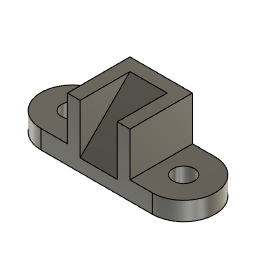
A2 (Autodesk Fusion 360 design; units mm, degrees)
Autodesk Fusion 360 part; units mm, degrees
sketch "Sketch2" plane through (0, 0, 0) normal (0, 0, 1) x (1, 0, 0)
  line L0 (57, -32) -> (-57, -32)
  line L1 (-57, 32) -> (57, 32)
  circle A0 centre (57, 0) radius 11
  circle A1 centre (-57, 0) radius 11
  arc A2 (-57, 32) -> (-57, -32) centre (-57, 0) ccw
  arc A3 (57, -32) -> (57, 32) centre (57, 0) ccw
  dimension "d15" = 114
  dimension "d17" = 32
  dimension "d18" = 32
  dimension "d19" = 22
  dimension "d20" = 22
  dimension "d21" = 114
  constraint horizontal L0
  constraint parallel L0 L1
  constraint concentric A0 A3
  constraint concentric A1 A2
  measures "d15" distance of L1.start L1.end
  measures "d17" radius of A3
  measures "d18" radius of A2
  measures "d19" diameter of A0
  measures "d20" diameter of A1
  measures "d21" distance of A0.centre A1.centre
extrude "Extrude1" add sketch "Sketch2" along normal blind 19
sketch "Sketch3" plane through (0, 0, 0) normal (0, 1, 0) x (1, 0, 0)
  line L0 (-30, 0) -> (34, 0)
  line L1 (34, 0) -> (34, -64)
  line L2 (34, -64) -> (-30, -64)
  line L3 (-30, -64) -> (-30, 0)
  dimension "d24" = 64
  dimension "d25" = 64
  constraint horizontal L0
  constraint vertical L1
  constraint horizontal L2
  constraint vertical L3
  measures "d24" distance of L0.start L0.end
  measures "d25" distance of L0.start L2.end
extrude "Extrude2" add sketch "Sketch3" along normal mid plane 64
shell "Shell1" thickness 13 removed faces 5 at (-8.6667, 32, 34) at (72.3041, 28.1031, 12.6667) at (12.6667, -32, 34) at (-77.5692, -24.5134, 12.6667) at (12.6667, -10.6667, 64)
sketch "Sketch4" plane through (0, 32, 0) normal (0, 1, 0) x (-1, 0, 0)
  line L0 (-21, 13) -> (-21, 64)
  line L1 (-21, 64) -> (-34, 64)
  line L2 (-34, 64) -> (-34, 19)
  line L3 (-34, 19) -> (-57, 19)
  line L4 (-57, 19) -> (-57, 0)
  line L5 (-57, 0) -> (57, 0)
  line L6 (57, 0) -> (57, 19)
  line L7 (57, 19) -> (30, 19)
  line L8 (30, 19) -> (30, 64)
  line L9 (30, 64) -> (17, 64)
  line L10 (17, 64) -> (17, 13)
  line L11 (17, 13) -> (-21, 13)
  line L12 (-21, 64) -> (17, 64)
  line L13 (17, 64) -> (17, 13)
  line L14 (17, 13) -> (-21, 13)
  line L15 (-21, 13) -> (-21, 64)
  constraint horizontal L12
  constraint vertical L13
  constraint horizontal L14
  constraint vertical L15
  constraint coincident L10.end L11.start
  constraint coincident L0.end L1.start
extrude "Extrude3" add sketch "Sketch4" against normal blind 13 contours L0 L10 L11 L12 L13 L14 L15
scale "Scale1" factor 0.887488 about (-17, -32, 64) bodies 1
sketch "Sketch8" plane through (16.7245, 0, 0) normal (-1, 0, 0) x (0, -1, 0)
  line L0 (-13.2619, 64) -> (-13.2619, 18.7381)
  line L1 (-13.2619, 18.7381) -> (32, 18.7381)
  line L2 (32, 18.7381) -> (32, 64)
  line L3 (32, 64) -> (-13.2619, 64)
  line L4 (-13.2619, 64) -> (32, 18.7381)
  line L5 (-13.2619, 18.7381) -> (-13.2619, 64)
  constraint coincident L0.start L3.end
  constraint coincident L1.end L2.start
  constraint coincident L0.end L1.start
extrude "Extrude6" add sketch "Sketch8" along normal blind 38 contours L0 L1 L4 L5
extrude "Extrude5" [rolled back] along distance 38 taper angle 0
